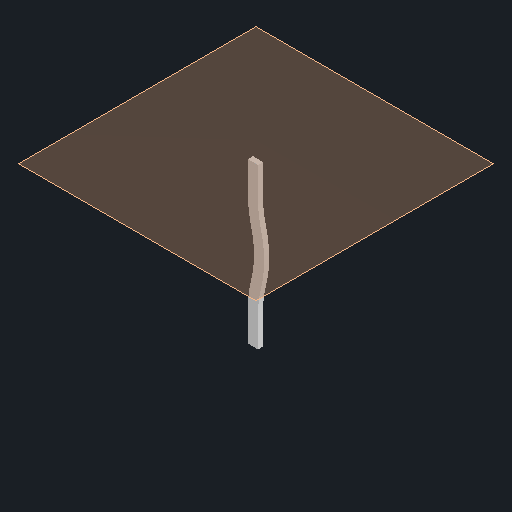
# Autodesk Inventor part: connector
Saved by Autodesk Inventor 2022 (Build 260153000, 153)
## iProperties
Created: 2023-02-02
Part Number: connector
Material: Generic
Document SubType Name: Modeling
Designer: erwin
Density: 1 g/cm^3
Appearance: Default
Author: erwin
Autodesk Inventor part; units mm, degrees
ref_plane "YZ Plane" through (0, 0, 0) normal (1, 0, 0) x (0, 1, 0)
ref_plane "XY Plane" through (0, 0, 0) normal (0, 0, 1) x (1, 0, 0)
sketch "Sketch1" plane through (0, 0, 0) normal (0, 0, 1) x (1, 0, 0)
  line L0 (0.9, 49.1) -> (0.9, 28.9) projected
  arc A0 (0.9, 49.1) -> (-0.9, 49.1) centre (0, 49.1) ccw projected
  line L1 (-0.9, 28.9) -> (-0.9, 49.1) projected
  arc A1 (-0.9, 28.9) -> (0.9, 28.9) centre (0, 28.9) ccw projected
  line L2 (0.9, 13.1) -> (0.9, -13.1) projected
  arc A2 (0.9, 13.1) -> (-0.9, 13.1) centre (0, 13.1) ccw projected
  line L3 (-0.9, -13.1) -> (-0.9, 13.1) projected
  arc A3 (-0.9, -13.1) -> (0.9, -13.1) centre (0, -13.1) ccw projected
  line L4 (0, 28.9) -> (0, 25.8465)
  arc A4 (0, 25.8465) -> (0.298, 23.4232) centre (10, 25.8465) ccw
  arc A5 (0.298, 18.5768) -> (0.298, 23.4232) centre (-9.4039, 21) ccw
  arc A6 (0.298, 18.5768) -> (0, 16.1535) centre (10, 16.1535) ccw
  line L5 (0, 16.1535) -> (0, 13.1)
  point P0 (0, 0)
  dimension "d0" = 10
  dimension "d1" = 10
  constraints: 6 point on circle, 4 end point, 4 tangent, 3 centre point, 2 collinear, 1 equal radius, 1 point on line, 1 vertical
  measures "d0" radius of A6
  measures "d1" radius of A5
ref_plane "Work Plane1" through (0, 28.9, 0) normal (0, 1, 0) x (-1, 0, 0)
sketch "Sketch2" plane through (0, 28.9, 0) normal (0, 1, 0) x (-1, 0, 0)
  line L0 (-0.5, 0) -> (0.5, 0)
  line L1 (0.5, 0) -> (0.5, -0.5)
  line L2 (0.5, -0.5) -> (-0.5, -0.5)
  line L3 (-0.5, -0.5) -> (-0.5, 0)
  point P0 (0, 0)
  point P1 (0, 0)
  dimension "d2" = 1
  dimension "d3" = 0.5
  constraints: 8 end point, 2 parallel, 1 coincident, 1 horizontal, 1 midpoint, 1 perpendicular
  measures "d2" distance of L1.end L2.end
  measures "d3" distance of L0.end L1.end
sweep "Sweep1" add profiles "Sketch2" path "Sketch1" path curves L4 A4 A5 A6 L5
body "Solid1"
